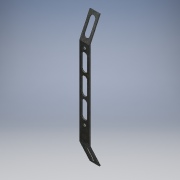
# Autodesk Inventor part: sled
Saved by Autodesk Inventor 2016 (Build 200138000, 138)
## iProperties
Created: 2015-11-15
Part Number: sled
Material: Steel
Document SubType Name: Modeling
Designer: Artur
Density: 7.85 g/cm^3
Appearance: Plate
Mass: 61.2667 g
Surface Area: 95.9585 cm^2
Volume: 7.80467 cm^3
Author: Artur
Autodesk Inventor part; units mm, degrees
ref_plane "XZ Plane" through (0, 0, 0) normal (0, 1, 0) x (-1, 0, 0)
ref_plane "XY Plane" through (0, 0, 0) normal (0, 0, 1) x (1, 0, 0)
sketch "Sketch1" plane through (0, 0, 0) normal (1, 0, 0) x (0, 1, 0)
  line L0 (0, 0) -> (0, -180)
  line L1 (0, -180) -> (21.1309, -225.3154)
  line L2 (21.1309, -225.3154) -> (22.9435, -224.4702)
  line L3 (22.9435, -224.4702) -> (2.2068, -180)
  line L4 (2.2068, -180) -> (2.2068, 0)
  line L5 (2.2068, 0) -> (22.9435, 44.4702)
  line L6 (22.9435, 44.4702) -> (21.1309, 45.3154)
  line L7 (0, 0) -> (21.1309, 45.3154)
  line L8 (0, 0) -> (67.9565, 0) construction
  dimension "d0" = 180
  dimension "d1" = 25
  dimension "d2" = 25
  dimension "d3" = 2
  dimension "d4" = 50
  dimension "d5" = 50
  constraints: 18 end point, 4 perpendicular, 2 parallel, 1 horizontal, 1 point on line, 1 vertical
  measures "d0" distance of L0.start L0.end
  measures "d1" angle of L0 L1
  measures "d2" angle of L0 L7
  measures "d3" distance between parallel lines of L7 L5
  measures "d4" distance from line of L0.start L6
  measures "d5" distance from line of L0.end L2
extrude "base" add sketch "Sketch1" along normal blind 20
sketch "Sketch2" plane through (0, 2.2068, 0) normal (0, 1, 0) x (1, 0, 0)
  circle A0 centre (10, 10) radius 3
  circle A1 centre (10, 146.5) radius 3
  line L0 (0, 0) -> (20, 0) construction
  line L1 (10, 0) -> (10, 23.1136) construction
  dimension "d8" = 6
  dimension "d9" = 6
  dimension "d10" = 10
  dimension "d11" = 136.5
  constraints: 2 centre point, 2 end point, 2 point on line, 1 midpoint, 1 vertical
  measures "d8" diameter of A0
  measures "d9" diameter of A1
  measures "d10" distance from line of L0 A0.centre
  measures "d11" distance of A1.centre A0.centre
extrude "holes" cut sketch "Sketch2" against normal blind 25
sketch "Sketch3" plane through (0, 2.2068, -180) normal (0, 0.9063, 0.4226) x (1, 0, 0)
  line L0 (0, 49.0674) -> (20, 49.0674) construction
  line L1 (10, 49.0674) -> (10, 4.5106) construction
  point P0 (0, -164.068)
  point P1 (10, 19.0674)
  dimension "d14" = 30
  constraints: 2 end point, 1 midpoint, 1 point on line, 1 vertical
  measures "d14" distance from line of point (10, 19.067) L0
hole "ballastHole_originalAtTheFront" [suppressed]
sketch "Sketch4" plane through (0, 2.2068, 0) normal (0, 1, 0) x (1, 0, 0)
  line L0 (0, 0) -> (20, 0) projected
  line L1 (0, 180) -> (20, 180) projected
  line L2 (10, 180) -> (10, 136)
  dimension "d30" = 44
  constraints: 2 end point, 1 coincident, 1 midpoint, 1 vertical
  measures "d30" distance of L2.start L2.end
hole "ballastHole" [suppressed]
sketch "Sketch5" plane through (0, 2.2068, -180) normal (0, 0.9063, 0.4226) x (1, 0, 0)
  line L0 (0, 0) -> (20, 0) construction
  line L1 (10, 0) -> (10, 49.0674) construction
  line L2 (0, 49.0674) -> (20, 49.0674) construction
  arc A0 (7, 9.5337) -> (13, 9.5337) centre (10, 9.5337) ccw
  line L3 (10, 9.5337) -> (7, 9.5337) construction
  line L4 (10, 9.5337) -> (13, 9.5337) construction
  line L5 (7, 9.5337) -> (7, 39.5337)
  line L6 (13, 9.5337) -> (13, 39.5337)
  arc A1 (13, 39.5337) -> (7, 39.5337) centre (10, 39.5337) ccw
  line L7 (10, 39.5337) -> (13, 39.5337) construction
  line L8 (10, 39.5337) -> (7, 39.5337) construction
  point P0 (0, -164.068)
  point P1 (10, 6.5337)
  dimension "d31" = 180
  dimension "d32" = 3
  dimension "d33" = 30
  dimension "d34" = 180
  dimension "d35" = 49.0674
  dimension "d36" = 6.5337
  constraints: 14 end point, 5 point on circle, 2 centre point, 2 midpoint, 2 vertical, 1 parallel, 1 perpendicular, 1 point on line
  measures "d31" angle of L3 L4
  measures "d32" distance of L3.end L3.start
  measures "d33" distance of L3.end L5.end
  measures "d34" angle of L8 L7
  measures "d35" distance between parallel lines of L2 L0
  measures "d36" distance from line of L0 point (10, 6.534)
extrude "Extrusion3" cut sketch "Sketch5" against normal blind 10
sketch "Sketch6" plane through (0, 22.9435, 44.4702) normal (0, 0.9063, -0.4226) x (1, 0, 0)
  line L0 (0, 0) -> (20, 0) construction
  line L1 (10, 0) -> (10, 50) construction
  line L2 (0, 50) -> (20, 50) construction
  arc A0 (4, 12.0337) -> (16, 12.0337) centre (10, 12.0337) ccw
  line L3 (10, 12.0337) -> (16, 12.0337) construction
  line L4 (10, 12.0337) -> (4, 12.0337) construction
  line L5 (4, 12.0337) -> (4, 37.0337)
  line L6 (16, 12.0337) -> (16, 37.0337)
  line L7 (0, 49.0674) -> (20, 49.0674) construction
  arc A1 (16, 37.0337) -> (4, 37.0337) centre (10, 37.0337) ccw
  line L8 (10, 37.0337) -> (16, 37.0337) construction
  line L9 (10, 37.0337) -> (4, 37.0337) construction
  point P0 (10, 6.0337)
  dimension "d39" = 180
  dimension "d40" = 6
  dimension "d41" = 25
  dimension "d42" = 49.0674
  dimension "d43" = 6.0337
  dimension "d44" = 180
  constraints: 14 end point, 5 point on circle, 2 centre point, 2 midpoint, 2 vertical, 1 parallel, 1 perpendicular, 1 point on line
  measures "d39" angle of L4 L3
  measures "d40" distance of L4.end L3.start
  measures "d41" distance of L4.end L5.end
  measures "d42" distance between parallel lines of L7 L0
  measures "d43" distance from line of L0 point (10, 6.034)
  measures "d44" angle of L9 L8
extrude "Extrusion4" cut sketch "Sketch6" against normal blind 10
sketch "Sketch7" plane through (0, 2.2068, 0) normal (0, 1, 0) x (1, 0, 0)
  line L0 (0, 0) -> (20, 0) construction
  line L1 (10, 0) -> (10, 180) construction
  line L2 (0, 180) -> (20, 180) construction
  arc A0 (4, 23) -> (16, 23) centre (10, 23) ccw
  line L3 (10, 23) -> (16, 23) construction
  line L4 (10, 23) -> (4, 23) construction
  line L5 (4, 23) -> (4, 48)
  line L6 (16, 23) -> (16, 48)
  circle A1 centre (10, 10) radius 3 construction
  line L7 (10, 13) -> (24.9558, 13) construction
  arc A2 (16, 48) -> (4, 48) centre (10, 48) ccw
  line L8 (10, 48) -> (4, 48) construction
  line L9 (10, 48) -> (16, 48) construction
  line L10 (10, 64.875) -> (4, 64.875) construction
  line L11 (10, 64.875) -> (16, 64.875) construction
  arc A3 (4, 64.875) -> (16, 64.875) centre (10, 64.875) ccw
  line L12 (4, 64.875) -> (4, 89.875)
  line L13 (16, 64.875) -> (16, 89.875)
  line L14 (10, 89.875) -> (4, 89.875) construction
  line L15 (10, 89.875) -> (16, 89.875) construction
  arc A4 (16, 89.875) -> (4, 89.875) centre (10, 89.875) ccw
  circle A5 centre (10, 146.5) radius 3 construction
  line L16 (10, 143.5) -> (28.9866, 143.5) construction
  line L17 (10, 106.75) -> (4, 106.75) construction
  line L18 (10, 106.75) -> (16, 106.75) construction
  arc A6 (4, 106.75) -> (16, 106.75) centre (10, 106.75) ccw
  line L19 (4, 106.75) -> (4, 131.75)
  line L20 (16, 106.75) -> (16, 131.75)
  line L21 (10, 131.75) -> (4, 131.75) construction
  line L22 (10, 131.75) -> (16, 131.75) construction
  arc A7 (16, 131.75) -> (4, 131.75) centre (10, 131.75) ccw
  point P0 (10, 17)
  point P1 (10, 58.875)
  point P2 (10, 100.75)
  point P3 (10, 7)
  dimension "d47" = 180
  dimension "d48" = 6
  dimension "d49" = 25
  dimension "d52" = 180
  dimension "d55" = 41.875
  dimension "d62" = 130.5
  dimension "d68" = 7
  dimension "d69" = 10
  constraints: 42 end point, 15 point on circle, 6 centre point, 4 horizontal, 4 point on line, 3 vertical, 2 midpoint, 1 collinear, 1 parallel, 1 tangent, 1 vertical alignment, 30 other
  measures "d47" angle of L3 L4
  measures "d48" distance of L4.end L3.start
  measures "d49" distance of L3.end L6.end
  measures "d52" angle of L9 L8
  measures "d55" distance of L3.start L10.start
  measures "d62" distance between parallel lines of L7 L16
  measures "d68" distance from line of L0 A1.end
  measures "d69" distance of L7.start L3.start
extrude "Extrusion5" cut sketch "Sketch7" against normal blind 10
ref_plane "Work Plane1" through (10, 22.9435, 44.4702) normal (1, 0, 0) x (0, 1, 0)
equation "\"d9\" = d8"
equation "\"d36\" = -d32 + 0.5 * d35 - 0.5 * d33"
equation "\"d43\" = -d40 + 0.5 * d42 - 0.5 * d41"
equation "\"d55\" = d49 + d51 + 2 * d48"
equation "\"d51\" = -1.5 * d48 - 0.75 * d49 + 0.25 * d62"
body "Solid1"
